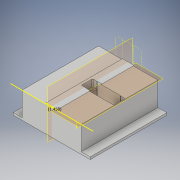
# Autodesk Inventor part: plateau_coulisseant
Saved by Autodesk Inventor 2018 (Build 220112000, 112)
## iProperties
Created: 2017-10-12
Part Number: plateau_coulisseant
Material: Generic
Document SubType Name: Modeling
Designer: liamg
Density: 1 g/cm^3
Appearance: Default
Author: liamg
Autodesk Inventor part; units mm, degrees
ref_plane "XZ Plane" through (0, 0, 0) normal (0, 1, 0) x (-1, 0, 0)
ref_plane "XY Plane" through (0, 0, 0) normal (0, 0, 1) x (1, 0, 0)
sketch "Sketch1" plane through (0, 0, 0) normal (0, 0, 1) x (1, 0, 0)
  line L0 (-9.963, 1.5182) -> (9.963, 1.5182) construction
  line L1 (9.963, 1.5182) -> (8.4447, 0) construction
  line L2 (18.795, 0) -> (8.4447, 0) construction
  line L3 (21.97, 0) -> (18.795, 0) construction
  line L4 (21.97, 0) -> (21.97, 26.825) construction
  line L5 (18.795, 30) -> (21.97, 26.825) construction
  line L6 (18.795, 30) -> (-18.795, 30) construction
  line L7 (-21.97, 26.825) -> (-18.795, 30) construction
  line L8 (-21.97, 26.825) -> (-21.97, 0) construction
  line L9 (-18.795, 0) -> (-21.97, 0) construction
  line L10 (-8.4447, 0) -> (-18.795, 0) construction
  line L11 (8.85, 30) -> (8.85, 2) construction
  line L12 (-9.85, 30) -> (-9.85, 2) construction
  line L13 (-8.4447, 0) -> (-9.963, 1.5182) construction
  point P0 (0, 0)
  point P1 (0, 0)
  constraints: 28 end point
sketch "Sketch2" plane through (0, 0, 0) normal (0, 0, 1) x (1, 0, 0)
  line L0 (24.03, 0.5901) -> (24.03, 6.9401) construction
  line L1 (38.1011, 0.5901) -> (38.1011, 6.9401) construction
  line L2 (40.9704, -9.5093) -> (40.9704, -4.8619) construction
  line L3 (40.9704, -9.5093) -> (47.3304, -9.5093) construction
  line L4 (40.9704, -10.7393) -> (47.3304, -10.7393) construction
  line L5 (40.9704, -37.5619) -> (40.9704, -10.7393) construction
  line L6 (39.9704, -37.5619) -> (1.7204, -37.5619) construction
  line L7 (0.7204, -10.7393) -> (0.7204, -37.5619) construction
  line L8 (0.7204, -4.8619) -> (0.7204, -9.5093) construction
  line L9 (0.9398, -10.7393) -> (-5.6396, -10.7393) construction
  line L10 (39.9704, -3.8619) -> (1.7204, -3.8619) construction
  line L11 (10.9571, -1.3619) -> (31.1204, -1.3619) construction
  line L12 (8.4344, 0) -> (50.3188, 0)
  line L13 (50.3188, 0) -> (50.3188, -44.2799)
  line L14 (50.3188, -44.2799) -> (0, -44.2799)
  line L15 (8.4344, 0) -> (8.3708, 0)
  line L16 (8.3708, 0) -> (9.8292, 1.4584)
  line L17 (9.8292, 1.4584) -> (0, 1.4584)
  line L18 (-8.4344, 0) -> (-50.3188, 0)
  line L19 (-50.3188, 0) -> (-50.3188, -44.2799)
  line L20 (-50.3188, -44.2799) -> (0, -44.2799)
  line L21 (-8.3708, 0) -> (-9.8292, 1.4584)
  line L22 (-9.8292, 1.4584) -> (0, 1.4584)
  line L23 (-8.3708, 0) -> (-8.4344, 0)
  point P0 (0, 0)
  point P1 (37.3029, -27.4984)
  dimension "d0" = 41.8844
  dimension "d1" = 45
  dimension "d2" = 45
  constraints: 48 end point, 4 horizontal, 1 perpendicular
  measures "d0" distance of L12.start L12.end
  measures "d1" angle of L15 L16
  measures "d2" angle of L17 L16
extrude "Extrusion1" add sketch "Sketch2" along normal blind 130
sketch "Sketch6" plane through (-9.8292, 1.4584, 0) normal (0, 1, 0) x (1, 0, 0)
  line L0 (1, -74.6503) -> (18.7, -74.6503) construction
  line L1 (19.7, -75.6503) -> (19.7, -113.9003) construction
  line L2 (0, -113.9003) -> (0, -75.6503) construction
  line L3 (-8.945, -124.6123) -> (-8.945, -5.3877) construction
  line L4 (-12.12, -5.3877) -> (-12.12, -124.6123) construction
  line L5 (28.645, -127.7873) -> (-8.945, -127.7873) construction
  line L6 (-12.12, -127.7873) -> (-8.945, -127.7873) construction
  line L7 (31.82, -124.6123) -> (31.82, -5.3877) construction
  line L8 (28.645, -2.2127) -> (-8.945, -2.2127) construction
  arc A0 (31.82, -5.3877) -> (28.645, -2.2127) centre (28.645, -5.3877) ccw construction
  arc A1 (-8.945, -2.2127) -> (-12.12, -5.3877) centre (-8.945, -5.3877) ccw construction
  arc A2 (28.645, -127.7873) -> (31.82, -124.6123) centre (28.645, -124.6123) ccw construction
  line L9 (0, -54.423) -> (0, -16.173) construction
  line L10 (50.6825, -54.6115) -> (12.4325, -54.6115)
  arc A3 (51.6825, -55.6115) -> (50.6825, -54.6115) centre (50.6825, -55.6115) ccw
  line L11 (51.6825, -73.3115) -> (51.6825, -55.6115)
  arc A4 (50.6825, -74.3115) -> (51.6825, -73.3115) centre (50.6825, -73.3115) ccw
  line L12 (12.4325, -74.3115) -> (50.6825, -74.3115)
  arc A5 (11.4325, -73.3115) -> (12.4325, -74.3115) centre (12.4325, -73.3115) ccw
  line L13 (11.4325, -55.6115) -> (11.4325, -73.3115)
  arc A6 (12.4325, -54.6115) -> (11.4325, -55.6115) centre (12.4325, -55.6115) ccw
  circle A7 centre (41.8325, -64.4615) radius 6.44 construction
  circle A8 centre (0, 0) radius 5.44 construction
  line L14 (51.6825, -54.9865) -> (58.0425, -54.9865) construction
  arc A9 (59.0425, -55.9865) -> (58.0425, -54.9865) centre (58.0425, -55.9865) ccw construction
  line L15 (59.0425, -72.9365) -> (59.0425, -55.9865) construction
  arc A10 (58.0425, -73.9365) -> (59.0425, -72.9365) centre (58.0425, -72.9365) ccw construction
  line L16 (51.6825, -73.9365) -> (58.0425, -73.9365) construction
  circle A11 centre (55.6202, -68.8215) radius 2.3 construction
  circle A12 centre (55.6202, -60.1015) radius 2.18 construction
  line L17 (11.6519, -54.9865) -> (5.0725, -54.9865) construction
  arc A13 (5.0725, -54.9865) -> (4.0725, -55.9865) centre (5.0725, -55.9865) ccw construction
  line L18 (4.0725, -72.9365) -> (4.0725, -55.9865) construction
  circle A14 centre (7.4948, -60.1015) radius 2.18 construction
  circle A15 centre (7.4948, -68.8215) radius 2.3 construction
  line L19 (5.0725, -73.9365) -> (11.6519, -73.9365) construction
  arc A16 (4.0725, -72.9365) -> (5.0725, -73.9365) centre (5.0725, -72.9365) ccw construction
  circle A17 centre (0, 0) radius 4.4768 construction
  line L20 (-5.3547, -0.1836) -> (-7.032, -1.2649) construction
  line L21 (-7.032, -1.2649) -> (-6.8876, -1.9) construction
  line L22 (-6.8876, -1.9) -> (-4.9076, -2.1498) construction
  line L23 (-7.0904, 0.8803) -> (-5.3567, -0.1081) construction
  line L24 (-6.9808, 1.5224) -> (-7.0904, 0.8803) construction
  line L25 (-5.0173, 1.8795) -> (-6.9808, 1.5224) construction
  line L26 (7.032, 1.2649) -> (6.8876, 1.9) construction
  line L27 (6.8876, 1.9) -> (4.9076, 2.1498) construction
  line L28 (5.3547, 0.1836) -> (7.032, 1.2649) construction
  line L29 (-7.032, -1.2649) -> (-6.8876, -1.9) construction
  line L30 (-6.9808, 1.5224) -> (-7.0904, 0.8803) construction
  line L31 (-5.3547, -0.1836) -> (-7.032, -1.2649) construction
  line L32 (-5.0173, 1.8795) -> (-6.9808, 1.5224) construction
  line L33 (60.148, 0) -> (-40.4896, 0) construction
  line L34 (9.85, -65) -> (23.9886, -65) construction
  point P0 (9.8292, 0)
  point P1 (-10.275, 0)
  constraints: 68 end point, 22 point on circle, 18 centre point, 1 coincident, 1 horizontal, 1 point on line
ref_plane "Work Plane1" through (8.3708, 0, 0) normal (0, 1, 0) x (1, 0, 0)
extrude "Extrusion2" cut sketch "Sketch6" against normal blind 37.2
sketch "Sketch7" plane through (8.3708, 0, 0) normal (0, 1, 0) x (1, 0, 0)
  point P0 (-8.3708, 0)
sketch "Sketch8" plane through (-9.8292, -35.7416, 0) normal (0, 1, 0) x (1, 0, 0)
  point P0 (9.8292, 0)
sketch "Sketch9" plane through (-9.8292, 1.4584, 0) normal (0, 1, 0) x (1, 0, 0)
  line L0 (1, -74.6503) -> (18.7, -74.6503) construction
  line L1 (19.7, -75.6503) -> (19.7, -113.9003) construction
  line L2 (0, -113.9003) -> (0, -75.6503) construction
  line L3 (-8.945, -124.6123) -> (-8.945, -5.3877) construction
  line L4 (-12.12, -5.3877) -> (-12.12, -124.6123) construction
  line L5 (28.645, -127.7873) -> (-8.945, -127.7873) construction
  line L6 (-12.12, -127.7873) -> (-8.945, -127.7873) construction
  line L7 (31.82, -124.6123) -> (31.82, -5.3877) construction
  line L8 (28.645, -2.2127) -> (-8.945, -2.2127) construction
  arc A0 (31.82, -5.3877) -> (28.645, -2.2127) centre (28.645, -5.3877) ccw construction
  arc A1 (-8.945, -2.2127) -> (-12.12, -5.3877) centre (-8.945, -5.3877) ccw construction
  arc A2 (28.645, -127.7873) -> (31.82, -124.6123) centre (28.645, -124.6123) ccw construction
  line L9 (0, -54.423) -> (0, -16.173) construction
  line L10 (50.6825, -54.6115) -> (12.4325, -54.6115) construction
  arc A3 (51.6825, -55.6115) -> (50.6825, -54.6115) centre (50.6825, -55.6115) ccw construction
  line L11 (51.6825, -73.3115) -> (51.6825, -55.6115)
  arc A4 (50.6825, -74.3115) -> (51.6825, -73.3115) centre (50.6825, -73.3115) ccw construction
  line L12 (12.4325, -74.3115) -> (50.6825, -74.3115) construction
  arc A5 (11.4325, -73.3115) -> (12.4325, -74.3115) centre (12.4325, -73.3115) ccw construction
  line L13 (11.4325, -55.6115) -> (11.4325, -73.3115)
  arc A6 (12.4325, -54.6115) -> (11.4325, -55.6115) centre (12.4325, -55.6115) ccw construction
  circle A7 centre (41.8325, -64.4615) radius 6.44 construction
  circle A8 centre (0, 0) radius 5.44 construction
  line L14 (51.6825, -54.9865) -> (58.0425, -54.9865)
  arc A9 (59.0425, -55.9865) -> (58.0425, -54.9865) centre (58.0425, -55.9865) ccw
  line L15 (59.0425, -72.9365) -> (59.0425, -55.9865)
  arc A10 (58.0425, -73.9365) -> (59.0425, -72.9365) centre (58.0425, -72.9365) ccw
  line L16 (51.6825, -73.9365) -> (58.0425, -73.9365)
  circle A11 centre (55.6202, -68.8215) radius 2.3 construction
  circle A12 centre (55.6202, -60.1015) radius 2.18 construction
  line L17 (11.6519, -54.9865) -> (5.0725, -54.9865)
  arc A13 (5.0725, -54.9865) -> (4.0725, -55.9865) centre (5.0725, -55.9865) ccw
  line L18 (4.0725, -72.9365) -> (4.0725, -55.9865)
  circle A14 centre (7.4948, -60.1015) radius 2.18 construction
  circle A15 centre (7.4948, -68.8215) radius 2.3 construction
  line L19 (5.0725, -73.9365) -> (11.6519, -73.9365)
  arc A16 (4.0725, -72.9365) -> (5.0725, -73.9365) centre (5.0725, -72.9365) ccw
  circle A17 centre (0, 0) radius 4.4768 construction
  line L20 (-5.3547, -0.1836) -> (-7.032, -1.2649) construction
  line L21 (-7.032, -1.2649) -> (-6.8876, -1.9) construction
  line L22 (-6.8876, -1.9) -> (-4.9076, -2.1498) construction
  line L23 (-7.0904, 0.8803) -> (-5.3567, -0.1081) construction
  line L24 (-6.9808, 1.5224) -> (-7.0904, 0.8803) construction
  line L25 (-5.0173, 1.8795) -> (-6.9808, 1.5224) construction
  line L26 (7.032, 1.2649) -> (6.8876, 1.9) construction
  line L27 (6.8876, 1.9) -> (4.9076, 2.1498) construction
  line L28 (5.3547, 0.1836) -> (7.032, 1.2649) construction
  line L29 (-7.032, -1.2649) -> (-6.8876, -1.9) construction
  line L30 (-6.9808, 1.5224) -> (-7.0904, 0.8803) construction
  line L31 (-5.3547, -0.1836) -> (-7.032, -1.2649) construction
  line L32 (-5.0173, 1.8795) -> (-6.9808, 1.5224) construction
  line L33 (60.148, 0) -> (-40.4896, 0) construction
  line L34 (9.85, -65) -> (23.9886, -65) construction
  line L35 (51.6825, -73.9365) -> (51.4631, -73.9365)
  arc A18 (50.6825, -74.3115) -> (51.6825, -73.3115) centre (50.6825, -73.3115) ccw construction
  line L36 (51.6825, -54.9865) -> (51.4631, -54.9865)
  line L37 (51.6825, -55.6115) -> (51.6825, -73.3115) projected
  arc A19 (51.6825, -55.6115) -> (51.4631, -54.9865) centre (50.6825, -55.6115) ccw
  arc A20 (51.4631, -73.9365) -> (51.6825, -73.3115) centre (50.6825, -73.3115) ccw
  arc A21 (11.4325, -73.3115) -> (11.6519, -73.9365) centre (12.4325, -73.3115) ccw
  arc A22 (11.6519, -54.9865) -> (11.4325, -55.6115) centre (12.4325, -55.6115) ccw
  point P0 (9.8292, 0)
  point P1 (9.8292, 0)
  point P2 (-10.275, 0)
  constraints: 74 end point, 32 point on circle, 22 centre point, 5 coincident, 3 horizontal, 1 point on line
sketch "Sketch10" plane through (0, 0, 130) normal (0, 0, 1) x (1, 0, 0)
  line L0 (-70.4463, 0) -> (70.4463, 0) projected
  line L1 (9.8292, 1.4584) -> (-9.8292, 1.4584) projected
  point P0 (0, 0)
  dimension "d8" = 1.4584
  measures "d8" distance between parallel lines of L0 L1
extrude "Extrusion3" cut sketch "Sketch9" against normal blind 11.835
sketch "Sketch11" plane through (0, 0, 130) normal (0, 0, 1) x (1, 0, 0)
  line L0 (-4.7567, 1.4584) -> (-4.7567, -10.3766) projected
  line L1 (41.6339, 0) -> (41.6339, -10.3766) projected
  point P0 (0, 0)
sketch "Sketch12" plane through (-9.8292, -10.3766, 0) normal (0, 1, 0) x (1, 0, 0)
  point P0 (9.8292, 0)
sketch "Sketch13" plane through (-9.8292, -10.3766, 0) normal (0, 1, 0) x (1, 0, 0)
  point P0 (9.8292, 0)
sketch "Sketch14" plane through (-9.8292, -10.3766, 0) normal (0, 1, 0) x (1, 0, 0)
  line L0 (1, -74.6503) -> (18.7, -74.6503) construction
  line L1 (19.7, -75.6503) -> (19.7, -113.9003) construction
  line L2 (0, -113.9003) -> (0, -75.6503) construction
  line L3 (-8.945, -124.6123) -> (-8.945, -5.3877) construction
  line L4 (-12.12, -5.3877) -> (-12.12, -124.6123) construction
  line L5 (28.645, -127.7873) -> (-8.945, -127.7873) construction
  line L6 (-12.12, -127.7873) -> (-8.945, -127.7873) construction
  line L7 (31.82, -124.6123) -> (31.82, -5.3877) construction
  line L8 (28.645, -2.2127) -> (-8.945, -2.2127) construction
  arc A0 (31.82, -5.3877) -> (28.645, -2.2127) centre (28.645, -5.3877) ccw construction
  arc A1 (-8.945, -2.2127) -> (-12.12, -5.3877) centre (-8.945, -5.3877) ccw construction
  arc A2 (28.645, -127.7873) -> (31.82, -124.6123) centre (28.645, -124.6123) ccw construction
  line L9 (0, -54.423) -> (0, -16.173) construction
  line L10 (50.6825, -54.6115) -> (12.4325, -54.6115) construction
  arc A3 (51.6825, -55.6115) -> (50.6825, -54.6115) centre (50.6825, -55.6115) ccw construction
  line L11 (51.6825, -73.3115) -> (51.6825, -55.6115) construction
  arc A4 (50.6825, -74.3115) -> (51.6825, -73.3115) centre (50.6825, -73.3115) ccw construction
  line L12 (12.4325, -74.3115) -> (50.6825, -74.3115) construction
  arc A5 (11.4325, -73.3115) -> (12.4325, -74.3115) centre (12.4325, -73.3115) ccw construction
  line L13 (11.4325, -55.6115) -> (11.4325, -73.3115) construction
  arc A6 (12.4325, -54.6115) -> (11.4325, -55.6115) centre (12.4325, -55.6115) ccw construction
  circle A7 centre (41.8325, -64.4615) radius 6.44 construction
  circle A8 centre (0, 0) radius 5.44 construction
  line L14 (51.6825, -54.9865) -> (58.0425, -54.9865) construction
  arc A9 (59.0425, -55.9865) -> (58.0425, -54.9865) centre (58.0425, -55.9865) ccw construction
  line L15 (59.0425, -72.9365) -> (59.0425, -55.9865) construction
  arc A10 (58.0425, -73.9365) -> (59.0425, -72.9365) centre (58.0425, -72.9365) ccw construction
  line L16 (51.6825, -73.9365) -> (58.0425, -73.9365) construction
  circle A11 centre (55.6202, -68.8215) radius 2.3
  circle A12 centre (55.6202, -60.1015) radius 2.18
  line L17 (11.6519, -54.9865) -> (5.0725, -54.9865) construction
  arc A13 (5.0725, -54.9865) -> (4.0725, -55.9865) centre (5.0725, -55.9865) ccw construction
  line L18 (4.0725, -72.9365) -> (4.0725, -55.9865) construction
  circle A14 centre (7.4948, -60.1015) radius 2.18
  circle A15 centre (7.4948, -68.8215) radius 2.3
  line L19 (5.0725, -73.9365) -> (11.6519, -73.9365) construction
  arc A16 (4.0725, -72.9365) -> (5.0725, -73.9365) centre (5.0725, -72.9365) ccw construction
  circle A17 centre (0, 0) radius 4.4768 construction
  line L20 (-5.3547, -0.1836) -> (-7.032, -1.2649) construction
  line L21 (-7.032, -1.2649) -> (-6.8876, -1.9) construction
  line L22 (-6.8876, -1.9) -> (-4.9076, -2.1498) construction
  line L23 (-7.0904, 0.8803) -> (-5.3567, -0.1081) construction
  line L24 (-6.9808, 1.5224) -> (-7.0904, 0.8803) construction
  line L25 (-5.0173, 1.8795) -> (-6.9808, 1.5224) construction
  line L26 (7.032, 1.2649) -> (6.8876, 1.9) construction
  line L27 (6.8876, 1.9) -> (4.9076, 2.1498) construction
  line L28 (5.3547, 0.1836) -> (7.032, 1.2649) construction
  line L29 (-7.032, -1.2649) -> (-6.8876, -1.9) construction
  line L30 (-6.9808, 1.5224) -> (-7.0904, 0.8803) construction
  line L31 (-5.3547, -0.1836) -> (-7.032, -1.2649) construction
  line L32 (-5.0173, 1.8795) -> (-6.9808, 1.5224) construction
  line L33 (60.148, 0) -> (-40.4896, 0) construction
  line L34 (9.85, -65) -> (23.9886, -65) construction
  line L35 (51.6825, -73.9365) -> (51.4631, -73.9365) construction
  arc A18 (50.6825, -74.3115) -> (51.6825, -73.3115) centre (50.6825, -73.3115) ccw construction
  line L36 (51.6825, -54.9865) -> (51.4631, -54.9865) construction
  line L37 (51.6825, -55.6115) -> (51.6825, -73.3115) construction
  arc A19 (51.6825, -55.6115) -> (51.4631, -54.9865) centre (50.6825, -55.6115) ccw construction
  arc A20 (51.4631, -73.9365) -> (51.6825, -73.3115) centre (50.6825, -73.3115) ccw construction
  arc A21 (11.4325, -73.3115) -> (11.6519, -73.9365) centre (12.4325, -73.3115) ccw construction
  arc A22 (11.6519, -54.9865) -> (11.4325, -55.6115) centre (12.4325, -55.6115) ccw construction
  point P0 (9.8292, 0)
  point P1 (9.8292, 0)
  point P2 (9.8292, 0)
  point P3 (-10.275, 0)
  constraints: 76 end point, 34 point on circle, 23 centre point, 5 coincident, 3 horizontal, 1 point on line
extrude "Extrusion4" cut sketch "Sketch14" against normal blind 11.835
sketch "Sketch15" plane through (50.3188, -44.2799, 0) normal (1, 0, 0) x (0, 0, -1)
  line L0 (0, 0) -> (-130, 0) projected
  line L1 (0, 44.2799) -> (0, 0) projected
  line L2 (-130, 0) -> (0, 0)
  line L3 (0, 0) -> (0, 4)
  line L4 (0, 4) -> (-130, 4)
  line L5 (-130, 4) -> (-130, 0)
  dimension "d13" = 4
  constraints: 8 end point, 2 parallel, 1 horizontal, 1 perpendicular, 1 point on line
  measures "d13" distance of L3.end L2.end
extrude "Extrusion5" add sketch "Sketch15" along normal blind 15
mirror "Mirror1" about plane through (0, 0, 0) normal (1, 0, 0) of "Extrusion5"
sketch "Sketch16" plane through (-50.3188, 0, 0) normal (-1, 0, 0) x (0, 0, 1)
  line L0 (55.6115, -10.3766) -> (55.6115, -35.7416) construction
  line L1 (73.3115, -10.3766) -> (73.3115, -35.7416) construction
  line L2 (55.6115, -35.7416) -> (73.3115, -35.7416) construction
  line L3 (55.6115, -25.7416) -> (73.3115, -25.7416) construction
  line L4 (59.8845, -25.6737) -> (69.0385, -25.6737)
  line L5 (69.0385, -25.6737) -> (69.0385, -29.6737)
  line L6 (69.0385, -29.6737) -> (59.8845, -29.6737)
  line L7 (59.8845, -29.6737) -> (59.8845, -25.6737)
  line L8 (59.8845, -25.6737) -> (69.0385, -29.6737) construction
  line L9 (69.0385, -25.6737) -> (59.8845, -29.6737) construction
  point P0 (0, 0)
  point P1 (64.4615, -25.7416)
  point P2 (64.4615, -27.6737)
  dimension "d16" = 10
  dimension "d17" = 4
  constraints: 14 end point, 3 midpoint, 2 parallel, 2 perpendicular, 2 point on line, 1 horizontal
  measures "d16" distance between parallel lines of L2 L3
  measures "d17" distance of L4.end L5.end
extrude "Extrusion6" cut sketch "Sketch16" against normal blind 59.45
body "Solid1"
